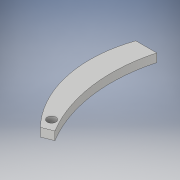
# Autodesk Inventor part: Gripper Arm
Saved by Autodesk Inventor 2018 (Build 220112000, 112)
## iProperties
Created: 2017-07-17
Part Number: Gripper Arm
Material: Generic
Document SubType Name: Modeling
Designer: James
Density: 1 g/cm^3
Appearance: Default
Author: James
Autodesk Inventor part; units mm, degrees
ref_plane "YZ Plane" through (0, 0, 0) normal (1, 0, 0) x (0, 1, 0)
ref_plane "XZ Plane" through (0, 0, 0) normal (0, 1, 0) x (-1, 0, 0)
ref_plane "XY Plane" through (0, 0, 0) normal (0, 0, 1) x (1, 0, 0)
sketch "Sketch3" plane through (0, 0, 0) normal (0, 1, 0) x (-1, 0, 0)
  arc A0 (19.5144, -87.8589) -> (0, 0) centre (-61.2135, -59.6928) ccw
  line L0 (19.5144, -87.8589) -> (4.5144, -87.8589)
  arc A1 (4.5144, -87.8589) -> (-7.4674, -2.9272) centre (-100.0611, -59.3009) ccw
  line L1 (-7.4674, -2.9272) -> (0, 0)
  dimension "d12" = 90
  dimension "d13" = 15
  constraints: 4 end point, 4 point on circle, 2 centre point, 1 horizontal
  measures "d12" distance of L1.end L0.start
  measures "d13" distance of L0.start L0.end
extrude "Extrusion2" add sketch "Sketch3" along normal blind 6
sketch "Sketch4" plane through (0, 6, 0) normal (0, 1, 0) x (1, 0, 0)
  circle A0 centre (-0.799, 8.7568) radius 2.1365
  point P0 (0, 0)
  constraints: 1 centre point
hole "Hole2" at (-0.799, 6, -8.7568) direction (0, -1, 0) diameter 6.25 depth 10 tip angle 118
body "Solid2"
